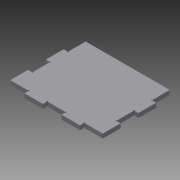
# Autodesk Inventor part: cajon lat grande
Saved by Autodesk Inventor 2015 (Build 190159000, 159)
## iProperties
Created: 2016-01-27
Part Number: cajon lat grande
Material: Generic
Document SubType Name: Modeling
Designer: iberopuebla
Density: 1 g/cm^3
Appearance: Default
Author: iberopuebla
Autodesk Inventor part; units mm, degrees
ref_plane "YZ Plane" through (0, 0, 0) normal (1, 0, 0) x (0, 1, 0)
ref_plane "XZ Plane" through (0, 0, 0) normal (0, 1, 0) x (-1, 0, 0)
ref_plane "XY Plane" through (0, 0, 0) normal (0, 0, 1) x (1, 0, 0)
sketch "Sketch1" plane through (0, 0, 0) normal (0, 0, 1) x (1, 0, 0)
  line L0 (195, 300) -> (18, 300)
  line L1 (78, -2.5) -> (78, -18)
  line L2 (156, -2.5) -> (156, -18)
  line L3 (78, -18) -> (156, -18)
  line L4 (158.5, 0) -> (195, 0)
  line L5 (0, 0) -> (0, 75)
  line L6 (0, 150) -> (0, 225)
  line L7 (18, 300) -> (18, 227.5)
  line L8 (18, 147.5) -> (18, 77.5)
  line L9 (0, 0) -> (75.5, 0)
  arc A0 (15.5, 225) -> (18, 227.5) centre (18, 225) ccw
  line L10 (0, 225) -> (15.5, 225)
  arc A1 (18, 147.5) -> (15.5, 150) centre (18, 150) ccw
  line L11 (0, 150) -> (15.5, 150)
  arc A2 (15.5, 75) -> (18, 77.5) centre (18, 75) ccw
  line L12 (0, 75) -> (15.5, 75)
  arc A3 (78, -2.5) -> (75.5, 0) centre (78, 0) ccw
  arc A4 (158.5, 0) -> (156, -2.5) centre (156, 0) ccw
  line L13 (390, 150) -> (374.5, 150)
  arc A5 (374.5, 150) -> (372, 147.5) centre (372, 150) ccw
  line L14 (390, 225) -> (374.5, 225)
  line L15 (390, 150) -> (390, 225)
  arc A6 (372, 227.5) -> (374.5, 225) centre (372, 225) ccw
  line L16 (372, 147.5) -> (372, 77.5)
  line L17 (372, 300) -> (372, 227.5)
  line L18 (312, -2.5) -> (312, -18)
  line L19 (234, -2.5) -> (234, -18)
  line L20 (312, -18) -> (234, -18)
  line L21 (390, 75) -> (374.5, 75)
  line L22 (390, 0) -> (390, 75)
  line L23 (390, 0) -> (314.5, 0)
  arc A7 (314.5, 0) -> (312, -2.5) centre (312, 0) ccw
  arc A8 (234, -2.5) -> (231.5, 0) centre (234, 0) ccw
  arc A9 (372, 77.5) -> (374.5, 75) centre (372, 75) ccw
  line L24 (195, 300) -> (372, 300)
  line L25 (231.5, 0) -> (195, 0)
  dimension "d0" = 78
  dimension "d1" = 78
  dimension "d2" = 300
  dimension "d3" = 5
  dimension "d4" = 18
  dimension "d5" = 5
  dimension "d6" = 15.5
  dimension "d7" = 5
  dimension "d8" = 18
  dimension "d9" = 15.5
  dimension "d10" = 5
  dimension "d11" = 5
  dimension "d12" = 18
  dimension "d13" = 18
  dimension "d14" = 78
  dimension "d15" = 75
  dimension "d16" = 75
  dimension "d17" = 75
  constraints: 52 end point, 22 point on circle, 10 centre point, 6 horizontal, 4 coincident, 4 vertical, 2 horizontal alignment, 2 perpendicular, 1 parallel, 1 vertical alignment, 1 other
  measures "d0" distance between parallel lines of L2 L1
  measures "d1" distance between parallel lines of L5 L1
  measures "d2" distance from line of L0 point (0, 0)
  measures "d3" diameter of A0
  measures "d4" distance from line of L7 L6.end
  measures "d5" diameter of A1
  measures "d6" distance of L6.start L11.end
  measures "d7" diameter of A2
  measures "d8" distance of A2.centre L5.end
  measures "d9" distance of L5.end L12.end
  measures "d10" diameter of A3
  measures "d11" diameter of A4
  measures "d12" distance from line of L2.end L4
  measures "d13" distance of L2.end A4.centre
  measures "d14" distance of A3.centre A4.centre
  measures "d15" distance between parallel lines of L0 L10
  measures "d16" distance of L6.start L6.end
  measures "d17" distance between parallel lines of L12 L11
extrude "Extrusion1" add sketch "Sketch1" along normal blind 18
body "Solid1"
